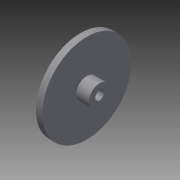
# Autodesk Inventor part: 知能ロボコンアルミギア１０３Ｃ
Saved by Autodesk Inventor 2013 (Build 170138000, 138)
## iProperties
Created: 2014-05-31
Part Number: 知能ロボコンアルミギア１０３Ｃ
Material: 一般
Document SubType Name: Modeling
Designer: horumo136
Density: 1 g/cm^3
Author: horumo136
Autodesk Inventor part; units mm, degrees
ref_plane "YZ Plane" through (0, 0, 0) normal (1, 0, 0) x (0, 1, 0)
ref_plane "XZ Plane" through (0, 0, 0) normal (0, 1, 0) x (-1, 0, 0)
ref_plane "XY Plane" through (0, 0, 0) normal (0, 0, 1) x (1, 0, 0)
sketch "スケッチ1" plane through (0, 0, 0) normal (1, 0, 0) x (0, 1, 0)
  circle A0 centre (0, 0) radius 1
  circle A1 centre (0, 0) radius 2.5
  circle A2 centre (0, 0) radius 13
  dimension "d0" = 2
  dimension "d1" = 5
  dimension "d2" = 26
  constraints: 3 centre point, 3 coincident
  measures "d0" diameter of A0
  measures "d1" diameter of A1
  measures "d2" diameter of A2
extrude "押し出し1" add sketch "スケッチ1" along normal blind 3 contours A1
sketch "スケッチ2" plane through (0, 0, 0) normal (-1, 0, 0) x (0, 0, 1)
  circle A0 centre (0, 0) radius 1 projected
  circle A1 centre (0, 0) radius 2.5 projected
  circle A2 centre (0, 0) radius 10.5
  dimension "d5" = 21
  constraints: 1 centre point, 1 coincident
  measures "d5" diameter of A2
extrude "押し出し2" add sketch "スケッチ2" along normal blind 1.5 contours A1 | A2
